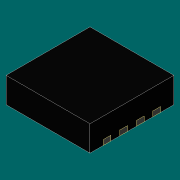
# Autodesk Inventor part: S3O8
Saved by Autodesk Inventor 2016 (Build 200138000, 138)
## iProperties
Created: 2015-11-05
Part Number: S3O8
Material: ABS Plastic
Document SubType Name: Modeling
Designer: Sawaiz
Density: 1.06 g/cm^3
Appearance: Smooth - Black
Author: Sawaiz
Autodesk Inventor part; units mm, degrees
ref_plane "YZ Plane" through (0, 0, 0) normal (1, 0, 0) x (0, 1, 0)
ref_plane "XZ Plane" through (0, 0, 0) normal (0, 1, 0) x (-1, 0, 0)
ref_plane "XY Plane" through (0, 0, 0) normal (0, 0, 1) x (1, 0, 0)
sketch "Sketch1" plane through (0, 0, 0) normal (0, 0, 1) x (1, 0, 0)
  line L0 (1.65, -1.65) -> (-1.65, -1.65)
  line L1 (-1.65, -1.65) -> (-1.65, 1.65)
  line L2 (-1.65, 1.65) -> (1.65, 1.65)
  line L3 (1.65, 1.65) -> (1.65, -1.65)
  line L4 (1.65, -1.65) -> (-1.65, 1.65) construction
  line L5 (-1.65, -1.65) -> (1.65, 1.65) construction
  point P0 (0, 0)
  dimension "d0" = 3.3
  dimension "d1" = 3.3
  constraints: 12 end point, 2 midpoint, 2 parallel, 1 horizontal, 1 perpendicular
  measures "d0" distance of L1.end L2.end
  measures "d1" distance of L0.end L1.end
extrude "Extrusion1" add sketch "Sketch1" along normal blind 1
sketch "Sketch2" plane through (0, 0, 0) normal (0, 0, -1) x (-1, 0, 0)
  line L0 (-1.65, -1.65) -> (1.65, -1.65) projected
  line L1 (1.65, -1.65) -> (1.65, 1.65) projected
  line L2 (1.65, 1.65) -> (-1.65, 1.65) projected
  line L3 (-1.65, 1.65) -> (-1.65, -1.65) projected
  line L4 (-1.125, -1.65) -> (-0.825, -1.65)
  line L5 (-0.825, -1.65) -> (-0.825, -1.15)
  line L6 (-0.825, -1.15) -> (-1.125, -1.15)
  line L7 (-1.125, -1.15) -> (-1.125, -1.65)
  line L8 (1.65, -1.65) -> (-1.65, -1.65) projected
  line L9 (-0.475, -1.65) -> (-0.175, -1.65)
  line L10 (-0.175, -1.65) -> (-0.175, -1.15)
  line L11 (-0.175, -1.15) -> (-0.475, -1.15)
  line L12 (-0.475, -1.15) -> (-0.475, -1.65)
  line L13 (0.175, -1.65) -> (0.475, -1.65)
  line L14 (0.475, -1.65) -> (0.475, -1.15)
  line L15 (0.475, -1.15) -> (0.175, -1.15)
  line L16 (0.175, -1.15) -> (0.175, -1.65)
  line L17 (0.825, -1.65) -> (1.125, -1.65)
  line L18 (1.125, -1.65) -> (1.125, -1.15)
  line L19 (1.125, -1.15) -> (0.825, -1.15)
  line L20 (0.825, -1.15) -> (0.825, -1.65)
  line L21 (1.125, 1.65) -> (-1.125, 1.65)
  line L22 (-1.125, 1.65) -> (-1.125, -0.45)
  line L23 (-1.125, -0.45) -> (1.125, -0.45)
  line L24 (1.125, -0.45) -> (1.125, 1.65)
  line L25 (0.825, 1.65) -> (0.475, 1.65)
  line L26 (0.475, 1.65) -> (0.475, 1.25)
  line L27 (0.475, 1.25) -> (0.825, 1.25)
  line L28 (0.825, 1.25) -> (0.825, 1.65)
  line L29 (0.175, 1.65) -> (-0.175, 1.65)
  line L30 (-0.175, 1.65) -> (-0.175, 1.25)
  line L31 (-0.175, 1.25) -> (0.175, 1.25)
  line L32 (0.175, 1.25) -> (0.175, 1.65)
  line L33 (-1.65, 1.65) -> (1.65, 1.65) projected
  line L34 (-0.475, 1.65) -> (-0.825, 1.65)
  line L35 (-0.825, 1.65) -> (-0.825, 1.25)
  line L36 (-0.825, 1.25) -> (-0.475, 1.25)
  line L37 (-0.475, 1.25) -> (-0.475, 1.65)
  line L38 (0, 1.65) -> (0, 1.25)
  point P0 (0, 0)
  dimension "d4" = 1.7
  dimension "d5" = 0.7
  dimension "d6" = 0.4
  dimension "d7" = 0.3
  dimension "d8" = 0.3
  dimension "d9" = 0.3
  dimension "d10" = 0.3
  dimension "d11" = 0.3
  dimension "d12" = 0.3
  dimension "d13" = 0.3
  dimension "d14" = 0.3
  dimension "d15" = 0.65
  dimension "d16" = 0.65
  dimension "d17" = 0.65
  dimension "d18" = 0.65
  dimension "d19" = 0.65
  constraints: 66 end point, 16 parallel, 14 point on line, 8 horizontal, 8 perpendicular, 2 midpoint, 1 collinear, 1 vertical
  measures "d4" distance between parallel lines of L23 L36
  measures "d5" distance between parallel lines of L6 L23
  measures "d6" distance between parallel lines of L34 L36
  measures "d7" distance between parallel lines of L7 L5
  measures "d8" distance between parallel lines of L12 L10
  measures "d9" distance between parallel lines of L14 L16
  measures "d10" distance between parallel lines of L18 L20
  measures "d11" distance between parallel lines of L22 L35
  measures "d12" distance between parallel lines of L30 L37
  measures "d13" distance between parallel lines of L26 L32
  measures "d14" distance between parallel lines of L24 L28
  measures "d15" distance between parallel lines of L12 L7
  measures "d16" distance between parallel lines of L16 L12
  measures "d17" distance between parallel lines of L20 L16
  measures "d18" distance between parallel lines of L22 L37
  measures "d19" distance between parallel lines of L32 L37
extrude "Extrusion2" cut sketch "Sketch2" against normal blind 0.2 contours L7 L6 L5 L0 | L2 L35 L36 L37 L30 L31 L32 L26 L27 L28 L24 L23 L22 | L12 L11 L10 L0 | L16 L15 L14 L0 | L20 L19 L18 L0
sketch "Sketch3" plane through (0, 0, 0) normal (0, 0, -1) x (-1, 0, 0)
  line L0 (0.175, 1.25) -> (0.175, 1.65) projected
  line L1 (-0.175, 1.25) -> (0.175, 1.25) projected
  line L2 (-0.175, 1.65) -> (-0.175, 1.25) projected
  line L3 (-0.475, 1.65) -> (-0.175, 1.65) projected
  line L4 (-0.475, 1.25) -> (-0.475, 1.65) projected
  line L5 (-0.825, 1.25) -> (-0.475, 1.25) projected
  line L6 (-0.825, 1.65) -> (-0.825, 1.25) projected
  line L7 (-1.125, 1.65) -> (-0.825, 1.65) projected
  line L8 (-1.125, -0.45) -> (-1.125, 1.65) projected
  line L9 (1.125, -0.45) -> (-1.125, -0.45) projected
  line L10 (1.125, 1.65) -> (1.125, -0.45) projected
  line L11 (0.825, 1.65) -> (1.125, 1.65) projected
  line L12 (0.825, 1.25) -> (0.825, 1.65) projected
  line L13 (0.475, 1.25) -> (0.825, 1.25) projected
  line L14 (0.475, 1.65) -> (0.475, 1.25) projected
  line L15 (0.175, 1.65) -> (0.475, 1.65) projected
  line L16 (-0.825, -1.65) -> (-1.125, -1.65) projected
  line L17 (-0.825, -1.15) -> (-0.825, -1.65) projected
  line L18 (-1.125, -1.15) -> (-0.825, -1.15) projected
  line L19 (-1.125, -1.65) -> (-1.125, -1.15) projected
  line L20 (-0.175, -1.65) -> (-0.475, -1.65) projected
  line L21 (-0.175, -1.15) -> (-0.175, -1.65) projected
  line L22 (-0.475, -1.15) -> (-0.175, -1.15) projected
  line L23 (-0.475, -1.65) -> (-0.475, -1.15) projected
  line L24 (0.475, -1.65) -> (0.175, -1.65) projected
  line L25 (0.475, -1.15) -> (0.475, -1.65) projected
  line L26 (0.175, -1.15) -> (0.475, -1.15) projected
  line L27 (0.175, -1.65) -> (0.175, -1.15) projected
  line L28 (1.125, -1.65) -> (0.825, -1.65) projected
  line L29 (1.125, -1.15) -> (1.125, -1.65) projected
  line L30 (0.825, -1.15) -> (1.125, -1.15) projected
  line L31 (0.825, -1.65) -> (0.825, -1.15) projected
  point P0 (0, 0)
extrude "Extrusion3" add sketch "Sketch3" against normal blind 0.2 separate body
body "Solid1"
body "Solid2"
